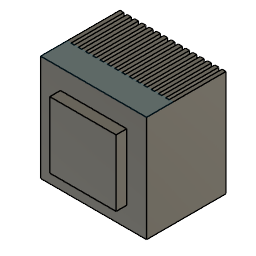
15_fin_ heat_sink (Autodesk Fusion 360 design; units mm, degrees)
Autodesk Fusion 360 part; units mm, degrees
sketch "Sketch1" plane through (0, 0, 0) normal (0, 1, 0) x (1, 0, 0)
  line L0 (0, 0) -> (25, 0)
  line L1 (25, 0) -> (25, -25)
  line L2 (25, -25) -> (0, -25)
  line L3 (0, -25) -> (0, 0)
  dimension "d1" = 25
  dimension "d2" = 25
  constraint coincident L0.start L3.end
  constraint horizontal L0
  constraint perpendicular L0 L1
  constraint perpendicular L1 L2
  constraint perpendicular L0 L3
  measures "d1" distance of L0.start L0.end
  measures "d2" distance of L0.end L1.end
extrude "Extrude1" add sketch "Sketch1" along normal blind 4
sketch "Sketch2" plane through (0, 4, 0) normal (0, 1, 0) x (-1, 0, 0)
  line L0 (0, 25) -> (-25, 25)
  line L1 (-25, 25) -> (-25, 0)
  line L2 (-25, 0) -> (0, 0)
  line L3 (0, 0) -> (0, 25)
  line L4 (-32.5, 32.5) -> (-32.5, -7.5)
  line L5 (-32.5, -7.5) -> (7.5, -7.5)
  line L6 (7.5, -7.5) -> (7.5, 32.5)
  line L7 (7.5, 32.5) -> (-32.5, 32.5)
  line L8 (-32.5, 32.5) -> (-12.5, 32.5)
  dimension "d6" = 40
  constraint perpendicular L2 L4
  constraint perpendicular L3 L5
  constraint perpendicular L0 L6
  constraint perpendicular L4 L7
  constraint midpoint L7 L8.end
  measures "d6" distance of L4.start L4.end
extrude "Extrude2" add sketch "Sketch2" along normal blind 10 contours L0 L1 L2 L3 | L4 L5 L6 L7 L8
sketch "Sketch3" plane through (0, 0, 32.5) normal (0, 0, 1) x (-1, 0, 0)
  line L0 (7.5, -4) -> (-32.5, -4)
  line L1 (-32.5, -4) -> (-32.5, -14)
  line L2 (-32.5, -14) -> (7.5, -14)
  line L3 (7.5, -14) -> (7.5, -4)
sketch "Sketch4" plane through (0, 0, 32.5) normal (0, 0, 1) x (-1, 0, 0)
  line L0 (7.5, -14) -> (7.5, -34)
  line L1 (7.5, -34) -> (5.5, -34)
  line L2 (5.5, -34) -> (5.5, -14)
  line L3 (5.5, -14) -> (7.5, -14)
  line L4 (3.28, -14) -> (3.28, -34)
  line L5 (3.28, -34) -> (1.28, -34)
  line L6 (1.28, -34) -> (1.28, -14)
  line L7 (-0.94, -14) -> (-0.94, -34)
  line L8 (-0.94, -34) -> (-2.94, -34)
  line L9 (-2.94, -34) -> (-2.94, -14)
  line L10 (-5.16, -14) -> (-5.16, -34)
  line L11 (-5.16, -34) -> (-7.16, -34)
  line L12 (-7.16, -34) -> (-7.16, -14)
  line L13 (-9.38, -14) -> (-9.38, -34)
  line L14 (-9.38, -34) -> (-11.38, -34)
  line L15 (-11.38, -34) -> (-11.38, -14)
  line L16 (-13.6, -14) -> (-13.6, -34)
  line L17 (-13.6, -34) -> (-15.6, -34)
  line L18 (-15.6, -34) -> (-15.6, -14)
  line L19 (-17.82, -14) -> (-17.82, -34)
  line L20 (-17.82, -34) -> (-19.82, -34)
  line L21 (-19.82, -34) -> (-19.82, -14)
  line L22 (-22.04, -14) -> (-22.04, -34)
  line L23 (-22.04, -34) -> (-24.04, -34)
  line L24 (-24.04, -34) -> (-24.04, -14)
  line L25 (-26.26, -14) -> (-26.26, -34)
  line L26 (-26.26, -34) -> (-28.26, -34)
  line L27 (-28.26, -34) -> (-28.26, -14)
  line L28 (-30.48, -14) -> (-30.48, -34)
  line L29 (-30.48, -34) -> (-32.48, -34)
  line L30 (-32.48, -34) -> (-32.48, -14)
  line L31 (7.5, -14) -> (-32.48, -14)
  line L32 (-32.48, -14) -> (7.5, -14)
  dimension "d11" = 20
  dimension "d12" = 2
  dimension "d15" = -4.22
  dimension "d16" = 0
  constraint vertical L0
  constraint perpendicular L0 L1
  constraint perpendicular L1 L2
  measures "d11" distance of L0.start L0.end
  measures "d12" distance of L0.end L1.end
sketch "Sketch5" plane through (0, 0, 32.5) normal (0, 0, 1) x (-1, 0, 0)
  line L0 (7.5, -14) -> (-32.5, -14)
  line L1 (7.5, -14) -> (7.5, -34)
  line L2 (7.5, -34) -> (6, -34)
  line L3 (6, -34) -> (6, -14)
  line L4 (7.5, -14) -> (6, -14)
  line L5 (4.75, -14) -> (4.75, -34)
  line L6 (3.25, -34) -> (3.25, -14)
  line L7 (4.75, -34) -> (3.25, -34)
  line L8 (2, -14) -> (2, -34)
  line L9 (0.5, -34) -> (0.5, -14)
  line L10 (2, -34) -> (0.5, -34)
  line L11 (-0.75, -14) -> (-0.75, -34)
  line L12 (-2.25, -34) -> (-2.25, -14)
  line L13 (-0.75, -34) -> (-2.25, -34)
  line L14 (-3.5, -14) -> (-3.5, -34)
  line L15 (-5, -34) -> (-5, -14)
  line L16 (-3.5, -34) -> (-5, -34)
  line L17 (-6.25, -14) -> (-6.25, -34)
  line L18 (-7.75, -34) -> (-7.75, -14)
  line L19 (-6.25, -34) -> (-7.75, -34)
  line L20 (-9, -14) -> (-9, -34)
  line L21 (-10.5, -34) -> (-10.5, -14)
  line L22 (-9, -34) -> (-10.5, -34)
  line L23 (-11.75, -14) -> (-11.75, -34)
  line L24 (-13.25, -34) -> (-13.25, -14)
  line L25 (-11.75, -34) -> (-13.25, -34)
  line L26 (-14.5, -14) -> (-14.5, -34)
  line L27 (-16, -34) -> (-16, -14)
  line L28 (-14.5, -34) -> (-16, -34)
  line L29 (-17.25, -14) -> (-17.25, -34)
  line L30 (-18.75, -34) -> (-18.75, -14)
  line L31 (-17.25, -34) -> (-18.75, -34)
  line L32 (-20, -14) -> (-20, -34)
  line L33 (-21.5, -34) -> (-21.5, -14)
  line L34 (-20, -34) -> (-21.5, -34)
  line L35 (-22.75, -14) -> (-22.75, -34)
  line L36 (-24.25, -34) -> (-24.25, -14)
  line L37 (-22.75, -34) -> (-24.25, -34)
  line L38 (-25.5, -14) -> (-25.5, -34)
  line L39 (-27, -34) -> (-27, -14)
  line L40 (-25.5, -34) -> (-27, -34)
  line L41 (-28.25, -14) -> (-28.25, -34)
  line L42 (-29.75, -34) -> (-29.75, -14)
  line L43 (-28.25, -34) -> (-29.75, -34)
  line L44 (-31, -14) -> (-31, -34)
  line L45 (-32.5, -34) -> (-32.5, -14)
  line L46 (-31, -34) -> (-32.5, -34)
  dimension "d19" = 20
  dimension "d22" = -2.75
  dimension "d23" = 0
  constraint horizontal L0
  constraint perpendicular L0 L1
  constraint perpendicular L1 L2
  constraint coincident L0 L3.end
  constraint perpendicular L0 L3
  measures "d19" distance of L0.start L1.end
extrude "Extrude4" add sketch "Sketch5" against normal blind 40
